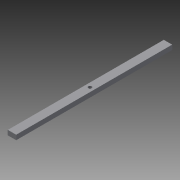
# Autodesk Inventor part: clip_base
Saved by Autodesk Inventor 2015 (Build 190159000, 159)
## iProperties
Created: 2017-10-02
Part Number: clip_base
Material: Generic
Document SubType Name: Modeling
Designer: Anshul
Density: 1 g/cm^3
Appearance: Default
Author: Anshul
Autodesk Inventor part; units mm, degrees
ref_plane "YZ Plane" through (0, 0, 0) normal (1, 0, 0) x (0, 1, 0)
ref_plane "XZ Plane" through (0, 0, 0) normal (0, 1, 0) x (-1, 0, 0)
ref_plane "XY Plane" through (0, 0, 0) normal (0, 0, 1) x (1, 0, 0)
sketch "Sketch1" plane through (0, 0, 0) normal (0, 1, 0) x (-1, 0, 0)
  circle A0 centre (0, 0) radius 6
  line L0 (6, 0) -> (15, 0)
  line L1 (15, 0) -> (15, -280)
  line L2 (15, -280) -> (-15, -280)
  line L3 (-15, -280) -> (-15, 0)
  line L4 (-15, 0) -> (-6, 0)
  line L5 (-15, 0) -> (-15, 280)
  line L6 (-15, 280) -> (15, 280)
  line L7 (15, 280) -> (15, 0)
  dimension "d0" = 12
  dimension "d1" = 15
  dimension "d2" = 280
  dimension "d3" = 30
  dimension "d4" = 280
  dimension "d5" = 30
  constraints: 16 end point, 4 perpendicular, 3 point on line, 2 point on circle, 1 centre point, 1 coincident, 1 horizontal
  measures "d0" diameter of A0
  measures "d1" distance of A0.centre L0.end
  measures "d2" distance of L0.end L1.end
  measures "d3" distance of L1.end L2.end
  measures "d4" distance of L3.end L5.end
  measures "d5" distance of L5.end L6.end
extrude "Extrusion1" add sketch "Sketch1" along normal blind 17 contours L0 L1 L2 L3 L4 A0 | A0 L4 L5 L6 L7 L0
body "Solid1"
